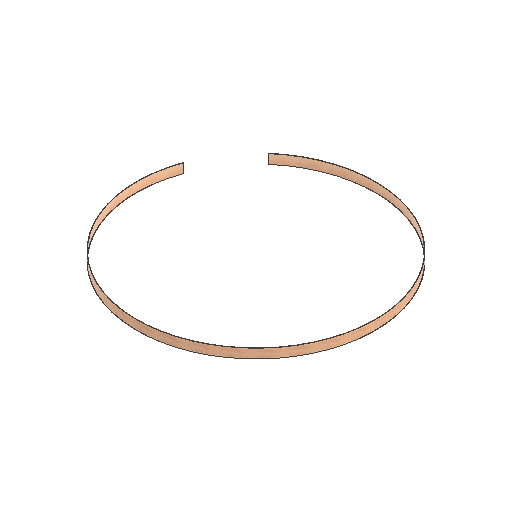
# Autodesk Inventor part: Edge Band - Platform D Outer
Saved by Autodesk Inventor 2021 (Build 250183000, 183)
## iProperties
Created: 2020-05-12
Part Number: Edge Band - Platform D Outer
Material: Wood (Birch)
Document SubType Name: Modeling
Designer: Dan Wikman
Density: 0.55 g/cm^3
Appearance: Birch - Natural Polished
Mass: 1619.28 g
Surface Area: 15317.6 cm^2
Volume: 2944.15 cm^3
Author: Dan Wikman
Autodesk Inventor part; units mm, degrees
ref_plane "YZ Plane" through (0, 0, 0) normal (1, 0, 0) x (0, 1, 0)
ref_plane "XZ Plane" through (0, 0, 0) normal (0, 1, 0) x (-1, 0, 0)
ref_plane "XY Plane" through (0, 0, 0) normal (0, 0, 1) x (1, 0, 0)
sketch "Sketch1" plane through (0, 0, 0) normal (0, 1, 0) x (-1, 0, 0)
  circle A0 centre (0, 0) radius 1275
  circle A1 centre (0, 0) radius 1279
  dimension "d0" = 2550
  dimension "d1" = 2558
  constraints: 2 centre point, 2 coincident
  measures "d0" diameter of A0
  measures "d1" diameter of A1
extrude "Extrusion1" add sketch "Sketch1" along normal blind 100
sketch "Sketch2" plane through (0, 0, 0) normal (0, -1, 0) x (1, 0, 0)
  line L0 (-601.6734, -761.7695) -> (-832.5638, -965.0384) projected
  line L1 (-1202.4006, -424.0965) -> (-929.1876, -282.72) projected
  circle A0 centre (0, 0) radius 1279 projected
  line L2 (-835.9402, -968.0108) -> (-832.9096, -965.3428)
  circle A1 centre (0, 0) radius 1275 projected
  line L3 (-1205.9873, -425.9525) -> (-1202.4006, -424.0965)
  constraints: 4 end point, 3 point on circle
extrude "Extrusion2" cut sketch "Sketch2" against normal blind 100 contours L3 A1 L2 A0 picked at (-1198.0722, -439.4962)
body "Solid1"
